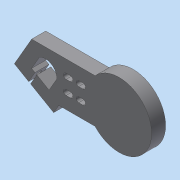
# Autodesk Inventor part: motormount3
Saved by Autodesk Inventor 2017 (Build 210142000, 142)
## iProperties
Created: 2015-12-12
Part Number: motormount3
Material: Generic
Document SubType Name: Modeling
Designer: JoshuaYuan
Density: 1 g/cm^3
Appearance: Default
Author: JoshuaYuan
Autodesk Inventor part; units mm, degrees
ref_plane "YZ Plane" through (0, 0, 0) normal (1, 0, 0) x (0, 1, 0)
ref_plane "XZ Plane" through (0, 0, 0) normal (0, 1, 0) x (-1, 0, 0)
ref_plane "XY Plane" through (0, 0, 0) normal (0, 0, 1) x (1, 0, 0)
sketch "Sketch1" plane through (0, 0, 0) normal (0, 0, 1) x (1, 0, 0)
  circle A0 centre (67.04, 0) radius 29.5
  line L0 (-5.2569, 9.1827) -> (-12.3689, -3.1356)
  line L1 (3.4689, -12.2796) -> (10.5809, 0.0387)
  arc A1 (10.5809, 0.0387) -> (-5.2569, 9.1827) centre (0.1701, 0.2946) ccw
  line L2 (-52.8871, 0) -> (121.4445, 0) projected
  line L3 (-12.2744, 19.8882) -> (-27.9826, -7.3193)
  line L4 (-27.9826, -7.3193) -> (-15.0193, -14.8037)
  line L5 (-12.2744, 19.8882) -> (45.2522, 19.8882)
  line L6 (0, -41.3) -> (0, 41.3) projected
  line L7 (-9.3043, -4.905) -> (-15.0193, -14.8037)
  line L8 (-13.2872, -15.8037) -> (-7.5722, -5.905)
  line L9 (-13.2872, -15.8037) -> (7.6526, -27.8933)
  line L10 (-12.3689, -3.1356) -> (-9.3043, -4.905)
  line L11 (-7.5722, -5.905) -> (3.4689, -12.2796)
  line L12 (7.6526, -27.8933) -> (12.2744, -19.8882)
  line L13 (12.2744, -19.8882) -> (45.2522, -19.8882)
  arc A2 (18.9859, 8.763) -> (18.9859, 3.937) centre (18.9859, 6.35) ccw
  arc A3 (22.7959, 3.937) -> (22.7959, 8.763) centre (22.7959, 6.35) ccw
  line L14 (18.9859, 8.763) -> (22.7959, 8.763)
  line L15 (22.7959, 3.937) -> (18.9859, 3.937)
  arc A4 (18.9859, -3.937) -> (18.9859, -8.763) centre (18.9859, -6.35) ccw
  arc A5 (22.7959, -8.763) -> (22.7959, -3.937) centre (22.7959, -6.35) ccw
  line L16 (18.9859, -3.937) -> (22.7959, -3.937)
  line L17 (22.7959, -8.763) -> (18.9859, -8.763)
  arc A6 (30.4159, 8.763) -> (30.4159, 3.937) centre (30.4159, 6.35) ccw
  arc A7 (34.2259, 3.937) -> (34.2259, 8.763) centre (34.2259, 6.35) ccw
  line L18 (30.4159, 8.763) -> (34.2259, 8.763)
  line L19 (34.2259, 3.937) -> (30.4159, 3.937)
  arc A8 (30.4159, -3.937) -> (30.4159, -8.763) centre (30.4159, -6.35) ccw
  arc A9 (34.2259, -8.763) -> (34.2259, -3.937) centre (34.2259, -6.35) ccw
  line L20 (30.4159, -3.937) -> (34.2259, -3.937)
  line L21 (34.2259, -8.763) -> (30.4159, -8.763)
  line L22 (5.3771, 9.3134) -> (-4.45, -7.7076) construction
  line L23 (7.9189, -4.572) -> (-7.9189, 4.572) construction
  point P0 (0, 0)
  point P1 (40.8299, 13.5382)
  point P2 (40.8299, -13.5382)
  dimension "d22" = 12.7
  dimension "d25" = 19.05
  dimension "d2" = 59
  dimension "d3" = 14.224
  dimension "d4" = 18.288
  dimension "d11" = 11.43
  dimension "d48" = 2
  dimension "d56" = 10.414
  dimension "d58" = 11.43
  dimension "d59" = 30
  dimension "d70" = 4.826
  dimension "d72" = 4.826
  dimension "d73" = 3.81
  dimension "d77" = 12.7
  dimension "d80" = 11.43
  dimension "d85" = 8.9
  dimension "d86" = 67.04
  dimension "d90" = 11.43
  constraints: 44 end point, 23 point on circle, 10 centre point, 7 perpendicular, 5 parallel, 4 horizontal, 4 point on line, 2 collinear, 2 tangent, 2 vertical, 1 midpoint, 1 symmetric about line, 30 other
  measures "d2" diameter of A0
  measures "d3" distance of L1.start L1.end
  measures "d4" distance of L0.end L1.start
  measures "d11" distance between parallel lines of L3 L0
  measures "d48" distance between parallel lines of L7 L8
  measures "d56" radius of A1
  measures "d58" distance between parallel lines of L4 L10
  measures "d59" angle of L2 L10
  measures "d70" diameter of A2
  measures "d72" diameter of A3
  measures "d73" distance of L15.start L15.end
  measures "d77" distance of L15.end L17.end
  measures "d80" distance of L15.end L19.end
  measures "d85" distance between parallel lines of L11 L23
  measures "d86" distance of point (0, 0) A0.centre
  measures "d90" distance between parallel lines of L12 L1
extrude "plate" add sketch "Sketch1" against normal blind 12.7 contours L2 A0 | A0 L2 | A0 L2 L1 A1 L6 L5 | L13 L12 L9 L6 L11 L1 L2 A0 | L6 A1 L0 L2 L3 L5 | L2 L0 L10 L7 L4 L3 | L9 L8 L11 L6 | L14 A3 L15 A2 | L16 A5 L17 A4 | L18 A7 L19 A6 | L20 A9 L21 A8
extrude "tension holes" cut sketch "Sketch1" against normal blind 25.4 contours L14 A3 L15 A2 | L16 A5 L17 A4 | L18 A7 L19 A6 | L20 A9 L21 A8
ref_plane "Work Plane1" through (14.1221, 4.6482, -12.7) normal (-0.8660254, 0.5, 0) x (0, 0, 1)
sketch "Sketch2" plane through (-12.2744, 19.8882, -12.7) normal (-0.8660254, 0.5, 0) x (0, 0, 1)
  line L0 (12.7, -19.9865) -> (0, -19.9865) projected
  line L1 (12.7, -31.4165) -> (0, -31.4165) projected
  line L2 (6.35, -19.9865) -> (6.35, -31.4165) construction
  circle A0 centre (6.35, -25.7015) radius 2.3813
  dimension "d60" = 4.7625
  constraints: 3 midpoint, 2 end point, 1 centre point
  measures "d60" diameter of A0
extrude "clamp screw" cut sketch "Sketch2" against normal through all
body "Solid1"
